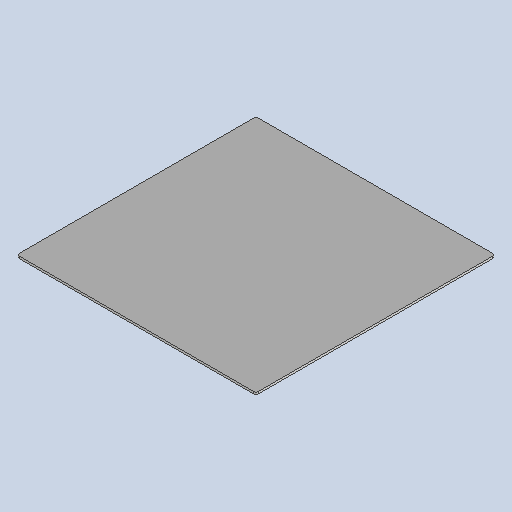
# Autodesk Inventor part: KND-1665 DrSysB CUP 1 01
Saved by Autodesk Inventor 2026.2 (Build 302298000, 298)
## iProperties
Created: 2025-06-24
Part Number: KND-1665 DrSysB CUP 1 01
Material: Stainless Steel
Document SubType Name: Sheet Metal
Designer: admin
Mass: 788.489 g
Surface Area: 1003.3 cm^2
Volume: 98.5611 cm^3
Density: 8 g/cm^3
Flat Pattern Width: 22.2 cm
Flat Pattern Length: 22.2 cm
Flat Pattern Area: 492.84 cm^2
Sheet Metal Rule: AISI304 2mm Die16
Sheet Metal Width: 222,000 mm
Sheet Metal Length: 222,000 mm
Sheet Metal Area: 49284,000 mm^2
Appearance: Default
Author: user
Autodesk Inventor part; units mm, degrees
ref_plane "YZ Plane" through (0, 0, 0) normal (1, 0, 0) x (0, 1, 0)
ref_plane "XZ Plane" through (0, 0, 0) normal (0, 1, 0) x (-1, 0, 0)
ref_plane "XY Plane" through (0, 0, 0) normal (0, 0, 1) x (1, 0, 0)
sketch "Sketch1" plane through (0, 0, 0) normal (0, 0, 1) x (1, 0, 0)
  line L0 (-111, -111) -> (111, -111)
  line L1 (111, -111) -> (111, 111)
  line L2 (111, 111) -> (-111, 111)
  line L3 (-111, 111) -> (-111, -111)
  line L4 (-111, -111) -> (111, 111) construction
  line L5 (111, -111) -> (-111, 111) construction
  point P0 (0, 0)
  dimension "d154" = 222
  dimension "d155" = 222
  measures "d154" distance of L1.end L2.end
  measures "d155" distance of L0.end L1.end
extrude "Plate5" add sketch "Sketch1" along normal blind 2
fillet "Corner Round1" radius 2 4 edges at (111, 111, 1) (-111, 111, 1) (-111, -111, 1) (111, -111, 1)
derived "KND-1401 DrSysB DIMentions 01.ipt"
body "Solid3"
